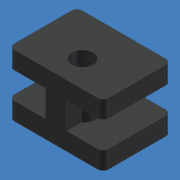
# Autodesk Inventor part: Servo Isolation Mounts1
Saved by Autodesk Inventor 2012 (Build 160160000, 160)
## iProperties
Shininess: 64.0
Length Units: 11269
Angle Units: 11279
Time Units: 11290
Mass Units: 11283
Length Display Precision: 3
Angle Display Precision: 2
Compacted: True
Part Number: Servo Isolation Mounts1
Document SubType Name: Modeling
Created: 2006-01-16
Material: ABS Plastic
Designer: Ed Sparks
Density: 1 g/cm^3
Density: 0.0
Volumn: 0.0
Area: 0.0
PropertySet Name: Model Information
Control State: 0
Master: False
Checked Out: False
Author: Ed Sparks
Autodesk Inventor part; units mm, degrees
ref_plane "YZ Plane" through (0, 0, 0) normal (1, 0, 0) x (0, 1, 0)
ref_plane "XZ Plane" through (0, 0, 0) normal (0, 1, 0) x (-1, 0, 0)
sketch "Sketch1" plane through (0, 0, 0) normal (0, 0, 1) x (1, 0, 0)
  line L0 (-4.435, 3.2) -> (4.435, 3.2)
  line L1 (4.435, 3.2) -> (4.435, -3.2)
  line L2 (4.435, -3.2) -> (-4.435, -3.2)
  line L3 (-4.435, -3.2) -> (-4.435, 3.2)
  line L4 (0, 0) -> (4.435, 0) construction
  line L5 (0, 0) -> (0, -3.2) construction
  line L6 (0, 0) -> (0, 3.2) construction
  line L7 (0, 0) -> (-4.435, 0) construction
  dimension "d0" = 8.87
  dimension "d1" = 6.4
  constraints: 16 end point, 5 perpendicular, 4 midpoint, 2 collinear, 2 parallel, 1 horizontal, 1 other
  measures "d0" distance of L0.start L0.end
  measures "d1" distance of L0.end L1.end
extrude "Extrusion1" add sketch "Sketch1" along normal mid plane 5.82
fillet "Fillet1" radius 0.5 4 edges at (4.435, -3.2, 0) (4.435, 3.2, 0) (-4.435, 3.2, 0) (-4.435, -3.2, 0)
sketch "Sketch2" plane through (0, 0, 2.91) normal (0, 0, 1) x (1, 0, 0)
  line L0 (-3.935, 3.2) -> (3.935, 3.2) projected
  circle A0 centre (0, -0.7) radius 1
  point P0 (0, 0)
  dimension "d5" = 3.9
  dimension "d6" = 2
  constraints: 1 centre point, 1 vertical alignment, 1 other
  measures "d5" distance from line of A0.centre L0
  measures "d6" diameter of A0
extrude "Extrusion2" cut sketch "Sketch2" against normal through all
ref_plane "Work Plane1" through (-3.935, -0.7, 2.91) normal (0, 1, 0) x (1, 0, 0)
sketch "Sketch5" plane through (-3.935, -0.7, 2.91) normal (0, 1, 0) x (1, 0, 0)
  line L0 (5.435, 1.66) -> (10.1042, 1.66)
  line L1 (10.1042, 1.66) -> (10.1042, 4.16)
  line L2 (10.1042, 4.16) -> (5.435, 4.16)
  line L3 (5.435, 4.16) -> (5.435, 1.66)
  line L4 (3.935, -1.746) -> (3.935, 6.402) projected
  line L5 (7.87, 0) -> (0, 0) projected
  line L6 (0, 5.82) -> (7.87, 5.82) projected
  dimension "d10" = 1.5
  dimension "d11" = 1.66
  dimension "d12" = 1.66
  constraints: 8 end point, 2 parallel, 1 horizontal, 1 perpendicular
  measures "d10" distance between parallel lines of L4 L3
  measures "d11" distance between parallel lines of L0 L5
  measures "d12" distance between parallel lines of L6 L2
revolve "Revolution1" cut sketch "Sketch5" angle 360 about axis through (0, -0.7, 2.91) along (0, 0, -1)
sketch "Sketch6" plane through (0, 0, 2.91) normal (0, 0, 1) x (1, 0, 0)
  circle A0 centre (0, -0.7) radius 1 projected
  line L0 (3.935, -3.2) -> (-3.935, -3.2) projected
  line L1 (-1, -0.7) -> (-1, -3.2)
  line L2 (1, -0.7) -> (1, -3.2)
  constraints: 4 end point, 2 point on circle, 2 point on line, 2 tangent, 1 parallel, 1 perpendicular
extrude "Extrusion3" add sketch "Sketch6" against normal through all contours L2 L0 L1 A0
body "Solid1"
